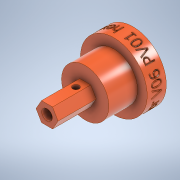
# Autodesk Inventor part: hexBushingForConnectorPiece
Saved by Autodesk Inventor 2022.2 (Build 262287000, 287)
## iProperties
Created: 2020-11-16
Part Number: hexBushingForConnectorPiece
Material: PC/ABS Plastic
Document SubType Name: Modeling
Designer: robst
Density: 0.357273 g/cm^3
Appearance: Smooth - Light Orange
Author: robst
Autodesk Inventor part; units mm, degrees
ref_plane "YZ Plane" through (0, 0, 0) normal (1, 0, 0) x (0, 1, 0)
ref_plane "XY Plane" through (0, 0, 0) normal (0, 0, 1) x (1, 0, 0)
sketch "Sketch1" plane through (0, 0, 0) normal (0, 0, 1) x (1, 0, 0)
  line L0 (7.3323, 0) -> (3.6662, -6.35)
  line L1 (3.6662, -6.35) -> (-3.6662, -6.35)
  line L2 (-3.6662, -6.35) -> (-7.3323, 0)
  line L3 (-7.3323, 0) -> (-3.6662, 6.35)
  line L4 (-3.6662, 6.35) -> (3.6662, 6.35)
  line L5 (3.6662, 6.35) -> (7.3323, 0)
  point P0 (0, 0)
  point P1 (0, 0)
  dimension "d0" = 12.7
  constraints: 12 end point, 1 coincident, 1 horizontal, 13 other
  measures "d0" distance between parallel lines of L1 L4
extrude "Extrusion1" add sketch "Sketch1" along normal mid plane 25.4
sketch "Sketch2" plane through (0, 0, -12.7) normal (0, 0, -1) x (-1, 0, 0)
  circle A0 centre (0, 0) radius 15.748
  dimension "d3" = 31.496
  constraints: 1 centre point, 1 coincident
  measures "d3" diameter of A0
extrude "Extrusion2" add sketch "Sketch2" along normal blind 19.05
sketch "Sketch3" plane through (0, 0, -31.75) normal (0, 0, -1) x (-1, 0, 0)
  circle A0 centre (0, 0) radius 22.225
  dimension "d6" = 44.45
  constraints: 1 centre point, 1 coincident
  measures "d6" diameter of A0
extrude "Extrusion3" add sketch "Sketch3" along normal blind 12.7
sketch "Sketch6" plane through (-3.6662, 6.35, 12.7) normal (0, 1, 0) x (1, 0, 0)
  line L0 (7.3323, 0) -> (0, 0) construction
  line L1 (3.6662, 0) -> (3.6662, 34.6111) construction
  line L2 (19.4142, 25.4) -> (-12.0818, 25.4) projected
  point P0 (3.6662, 12.7)
  point P1 (3.6662, 19.2024)
  dimension "d13" = 6.1976
  constraints: 2 end point, 1 midpoint, 1 point on line, 1 vertical
  measures "d13" distance from line of point (3.666, 19.202) L2
hole "Hole1" at (0, 6.35, -6.5024) direction (0, -1, 0) diameter 4.318 end through all clearance for "Hex Machine Screw" size "#6" standard "Ansi Unified Screw Threads"
sketch "Sketch7" plane through (0, 0, 12.7) normal (0, 0, 1) x (1, 0, 0)
  point P0 (0, 0)
  point P1 (0, 0)
  constraints: 1 coincident
hole "Hole2" at (0, 0, 12.7) direction (0, 0, -1) diameter 6.3246 depth 7.874 counterbore diameter 7.0891 counterbore depth 6.1239
ref_plane "Work Plane1" through (0, -22.225, -31.75) normal (0, 1, 0) x (-1, 0, 0)
sketch "Sketch8" plane through (0, -22.225, -31.75) normal (0, 1, 0) x (-1, 0, 0)
  line L0 (-22.225, -12.7) -> (22.225, -12.7) projected
  line L1 (-22.225, 0) -> (22.225, 0) projected
  line L2 (22.225, 0) -> (22.225, -12.7) construction
  line L3 (22.225, -6.35) -> (-22.225, -6.35) construction
  line L4 (-22.225, 0) -> (-22.225, -12.7) construction
  line L5 (63.482, -9.525) -> (64.2847, -9.525)
  line L6 (64.2847, -9.525) -> (64.2847, -6.808)
  spline S0 degree 2 poles (64.2847, -6.808) (64.2847, -6.4786) (64.3465, -5.9126) (64.4391, -5.7428) knots 0 0 0 1 2 2 2
  spline S1 degree 2 poles (64.4391, -5.7428) (64.5369, -5.5627) (64.8868, -5.3877) (65.1853, -5.3877) knots 0 0 0 1 2 2 2
  spline S2 degree 2 poles (65.1853, -5.3877) (65.4837, -5.3877) (66.1167, -5.7068) (66.4203, -5.9641) knots 0 0 0 1 2 2 2
  line L7 (66.4203, -5.9641) -> (66.4203, -9.525)
  line L8 (66.4203, -9.525) -> (67.223, -9.525)
  line L9 (67.223, -9.525) -> (67.223, -2.892)
  line L10 (67.223, -2.892) -> (66.4203, -2.892)
  line L11 (66.4203, -2.892) -> (66.4203, -5.29)
  spline S3 degree 2 poles (66.4203, -5.29) (66.0601, -4.9658) (65.3654, -4.6261) (64.9743, -4.6261) knots 0 0 0 1 2 2 2
  spline S4 degree 2 poles (64.9743, -4.6261) (64.2744, -4.6261) (63.482, -5.5524) (63.482, -6.4323) knots 0 0 0 1 2 2 2
  line L12 (63.482, -6.4323) -> (63.482, -9.525)
  spline S5 degree 2 poles (60.2864, -9.6331) (61.4288, -9.6331) (62.6844, -8.3517) (62.6844, -7.1682) knots 0 0 0 1 2 2 2
  spline S6 degree 2 poles (62.6844, -7.1682) (62.6844, -6.0052) (61.4648, -4.6261) (60.4819, -4.6261) knots 0 0 0 1 2 2 2
  spline S7 degree 2 poles (60.4819, -4.6261) (60.0394, -4.6261) (59.355, -4.8834) (59.1029, -5.1562) knots 0 0 0 1 2 2 2
  spline S8 degree 2 poles (59.1029, -5.1562) (58.8456, -5.4289) (58.5728, -6.2162) (58.5728, -6.7874) knots 0 0 0 1 2 2 2
  line L13 (58.5728, -6.7874) -> (58.5728, -7.2248)
  line L14 (58.5728, -7.2248) -> (61.8713, -7.2248)
  spline S9 degree 2 poles (61.8713, -7.2248) (61.8713, -8.0533) (61.0377, -8.9332) (60.2967, -8.9332) knots 0 0 0 1 2 2 2
  spline S10 degree 2 poles (60.2967, -8.9332) (60.0343, -8.9332) (59.5248, -8.8149) (59.319, -8.7222) knots 0 0 0 1 2 2 2
  spline S11 degree 2 poles (59.319, -8.7222) (59.1029, -8.6193) (58.8044, -8.4392) (58.7066, -8.3569) knots 0 0 0 1 2 2 2
  line L15 (58.7066, -8.3569) -> (58.6603, -8.3569)
  line L16 (58.6603, -8.3569) -> (58.6603, -9.2317)
  spline S12 degree 2 poles (58.6603, -9.2317) (58.7992, -9.2883) (59.2212, -9.453) (59.3859, -9.4993) knots 0 0 0 1 2 2 2
  spline S13 degree 2 poles (59.3859, -9.4993) (59.6174, -9.5662) (59.9982, -9.6331) (60.2864, -9.6331) knots 0 0 0 1 2 2 2
  spline S14 degree 2 poles (59.355, -6.6124) (59.3653, -6.2882) (59.4991, -5.8148) (59.6277, -5.6553) knots 0 0 0 1 2 2 2
  spline S15 degree 2 poles (59.6277, -5.6553) (59.7667, -5.4752) (60.2041, -5.2848) (60.5283, -5.2848) knots 0 0 0 1 2 2 2
  spline S16 degree 2 poles (60.5283, -5.2848) (60.8473, -5.2848) (61.295, -5.4752) (61.4802, -5.6605) knots 0 0 0 1 2 2 2
  spline S17 degree 2 poles (61.4802, -5.6605) (61.6603, -5.8509) (61.8456, -6.3088) (61.8713, -6.6124) knots 0 0 0 1 2 2 2
  line L17 (61.8713, -6.6124) -> (59.355, -6.6124)
  line L18 (54.0599, -9.525) -> (55.0428, -9.525)
  line L19 (55.0428, -9.525) -> (56.2006, -7.7342)
  line L20 (56.2006, -7.7342) -> (57.3893, -9.525)
  line L21 (57.3893, -9.525) -> (58.3001, -9.525)
  line L22 (58.3001, -9.525) -> (56.6483, -7.163)
  line L23 (56.6483, -7.163) -> (58.2847, -4.7599)
  line L24 (58.2847, -4.7599) -> (57.3018, -4.7599)
  line L25 (57.3018, -4.7599) -> (56.1491, -6.5353)
  line L26 (56.1491, -6.5353) -> (54.9707, -4.7599)
  line L27 (54.9707, -4.7599) -> (54.0599, -4.7599)
  line L28 (54.0599, -4.7599) -> (55.7014, -7.1116)
  line L29 (55.7014, -7.1116) -> (54.0599, -9.525)
  spline S18 degree 2 poles (49.0684, -7.5747) (49.0684, -8.0481) (49.4286, -8.7737) (49.7271, -9.0104) knots 0 0 0 1 2 2 2
  spline S19 degree 2 poles (49.7271, -9.0104) (50.0873, -9.2883) (50.9055, -9.525) (51.5539, -9.525) knots 0 0 0 1 2 2 2
  line L30 (51.5539, -9.525) -> (53.3755, -9.525)
  line L31 (53.3755, -9.525) -> (53.3755, -3.175)
  line L32 (53.3755, -3.175) -> (51.6928, -3.175)
  spline S20 degree 2 poles (51.6928, -3.175) (51.0135, -3.175) (50.3343, -3.2625) (50.0255, -3.4323) knots 0 0 0 1 2 2 2
  spline S21 degree 2 poles (50.0255, -3.4323) (49.6808, -3.6124) (49.3669, -4.2042) (49.3669, -4.6056) knots 0 0 0 1 2 2 2
  spline S22 degree 2 poles (49.3669, -4.6056) (49.3669, -5.0532) (49.8403, -5.7634) (50.2571, -5.9641) knots 0 0 0 1 2 2 2
  line L33 (50.2571, -5.9641) -> (50.2571, -5.9949)
  spline S23 degree 2 poles (50.2571, -5.9949) (49.6911, -6.1493) (49.0684, -6.9675) (49.0684, -7.5747) knots 0 0 0 1 2 2 2
  spline S24 degree 2 poles (49.9484, -7.6107) (49.9484, -7.2505) (50.1542, -6.7874) (50.4629, -6.6227) knots 0 0 0 1 2 2 2
  spline S25 degree 2 poles (50.4629, -6.6227) (50.6636, -6.5198) (51.1371, -6.4581) (51.5744, -6.4581) knots 0 0 0 1 2 2 2
  line L34 (51.5744, -6.4581) -> (52.5316, -6.4581)
  line L35 (52.5316, -6.4581) -> (52.5316, -8.8046)
  line L36 (52.5316, -8.8046) -> (51.8472, -8.8046)
  spline S26 degree 2 poles (51.8472, -8.8046) (51.2914, -8.8046) (50.6533, -8.7017) (50.4063, -8.537) knots 0 0 0 1 2 2 2
  spline S27 degree 2 poles (50.4063, -8.537) (50.1696, -8.3672) (49.9484, -7.9452) (49.9484, -7.6107) knots 0 0 0 1 2 2 2
  spline S28 degree 2 poles (50.2468, -4.7239) (50.2468, -4.4975) (50.4012, -4.1579) (50.571, -4.0601) knots 0 0 0 1 2 2 2
  spline S29 degree 2 poles (50.571, -4.0601) (50.7768, -3.9469) (51.276, -3.8954) (51.7237, -3.8954) knots 0 0 0 1 2 2 2
  line L37 (51.7237, -3.8954) -> (52.5316, -3.8954)
  line L38 (52.5316, -3.8954) -> (52.5316, -5.7531)
  line L39 (52.5316, -5.7531) -> (51.5744, -5.7531)
  spline S30 degree 2 poles (51.5744, -5.7531) (51.1782, -5.7531) (50.8026, -5.6707) (50.6019, -5.5421) knots 0 0 0 1 2 2 2
  spline S31 degree 2 poles (50.6019, -5.5421) (50.4063, -5.4186) (50.2468, -5.0224) (50.2468, -4.7239) knots 0 0 0 1 2 2 2
  line L40 (44.5864, -9.525) -> (45.3891, -9.525)
  line L41 (45.3891, -9.525) -> (45.3891, -9.0001)
  spline S32 degree 2 poles (45.3891, -9.0001) (45.7596, -9.3243) (46.4234, -9.6588) (46.8351, -9.6588) knots 0 0 0 1 2 2 2
  spline S33 degree 2 poles (46.8351, -9.6588) (47.1439, -9.6588) (47.6945, -9.453) (47.8952, -9.2317) knots 0 0 0 1 2 2 2
  spline S34 degree 2 poles (47.8952, -9.2317) (48.101, -9.0104) (48.3274, -8.3363) (48.3274, -7.8526) knots 0 0 0 1 2 2 2
  line L42 (48.3274, -7.8526) -> (48.3274, -4.7599)
  line L43 (48.3274, -4.7599) -> (47.5247, -4.7599)
  line L44 (47.5247, -4.7599) -> (47.5247, -7.4769)
  spline S35 degree 2 poles (47.5247, -7.4769) (47.5247, -7.8577) (47.468, -8.3569) (47.3703, -8.5421) knots 0 0 0 1 2 2 2
  spline S36 degree 2 poles (47.3703, -8.5421) (47.2725, -8.7274) (46.938, -8.8972) (46.6241, -8.8972) knots 0 0 0 1 2 2 2
  spline S37 degree 2 poles (46.6241, -8.8972) (46.3308, -8.8972) (45.667, -8.5627) (45.3891, -8.3209) knots 0 0 0 1 2 2 2
  line L45 (45.3891, -8.3209) -> (45.3891, -4.7599)
  line L46 (45.3891, -4.7599) -> (44.5864, -4.7599)
  line L47 (44.5864, -4.7599) -> (44.5864, -9.525)
  spline S38 degree 2 poles (42.1369, -9.6382) (42.6155, -9.6382) (43.444, -9.3809) (43.7167, -9.2368) knots 0 0 0 1 2 2 2
  line L48 (43.7167, -9.2368) -> (43.7167, -8.3363)
  line L49 (43.7167, -8.3363) -> (43.6755, -8.3363)
  spline S39 degree 2 poles (43.6755, -8.3363) (43.5726, -8.4186) (43.2947, -8.6142) (43.0632, -8.7222) knots 0 0 0 1 2 2 2
  spline S40 degree 2 poles (43.0632, -8.7222) (42.8625, -8.82) (42.3685, -8.9641) (42.1061, -8.9641) knots 0 0 0 1 2 2 2
  spline S41 degree 2 poles (42.1061, -8.9641) (41.9157, -8.9641) (41.4783, -8.8766) (41.3753, -8.8046) knots 0 0 0 1 2 2 2
  spline S42 degree 2 poles (41.3753, -8.8046) (41.2261, -8.7068) (41.0923, -8.4855) (41.0923, -8.2591) knots 0 0 0 1 2 2 2
  spline S43 degree 2 poles (41.0923, -8.2591) (41.0923, -7.9761) (41.4011, -7.6828) (41.7973, -7.585) knots 0 0 0 1 2 2 2
  spline S44 degree 2 poles (41.7973, -7.585) (41.9517, -7.549) (42.4457, -7.4461) (42.6567, -7.3895) knots 0 0 0 1 2 2 2
  spline S45 degree 2 poles (42.6567, -7.3895) (43.2021, -7.2299) (43.6961, -6.5713) (43.6961, -6.103) knots 0 0 0 1 2 2 2
  spline S46 degree 2 poles (43.6961, -6.103) (43.6961, -5.4546) (42.7236, -4.6467) (41.9208, -4.6467) knots 0 0 0 1 2 2 2
  spline S47 degree 2 poles (41.9208, -4.6467) (41.5246, -4.6467) (40.7218, -4.8423) (40.4491, -4.9915) knots 0 0 0 1 2 2 2
  line L50 (40.4491, -4.9915) -> (40.4491, -5.8509)
  line L51 (40.4491, -5.8509) -> (40.4903, -5.8509)
  spline S48 degree 2 poles (40.4903, -5.8509) (40.799, -5.6038) (41.5503, -5.3208) (41.9362, -5.3208) knots 0 0 0 1 2 2 2
  spline S49 degree 2 poles (41.9362, -5.3208) (42.3325, -5.3208) (42.8779, -5.6553) (42.8779, -5.9898) knots 0 0 0 1 2 2 2
  spline S50 degree 2 poles (42.8779, -5.9898) (42.8779, -6.2934) (42.5537, -6.5867) (42.1935, -6.6793) knots 0 0 0 1 2 2 2
  spline S51 degree 2 poles (42.1935, -6.6793) (42.0186, -6.7256) (41.576, -6.8183) (41.3342, -6.8749) knots 0 0 0 1 2 2 2
  spline S52 degree 2 poles (41.3342, -6.8749) (40.8093, -7.0087) (40.2741, -7.621) (40.2741, -8.1511) knots 0 0 0 1 2 2 2
  spline S53 degree 2 poles (40.2741, -8.1511) (40.2741, -8.4598) (40.516, -9.0053) (40.7527, -9.206) knots 0 0 0 1 2 2 2
  spline S54 degree 2 poles (40.7527, -9.206) (41.0048, -9.4169) (41.6481, -9.6382) (42.1369, -9.6382) knots 0 0 0 1 2 2 2
  line L52 (35.7869, -9.525) -> (36.5897, -9.525)
  line L53 (36.5897, -9.525) -> (36.5897, -6.808)
  spline S55 degree 2 poles (36.5897, -6.808) (36.5897, -6.4786) (36.6514, -5.9126) (36.7441, -5.7428) knots 0 0 0 1 2 2 2
  spline S56 degree 2 poles (36.7441, -5.7428) (36.8418, -5.5627) (37.1918, -5.3877) (37.4902, -5.3877) knots 0 0 0 1 2 2 2
  spline S57 degree 2 poles (37.4902, -5.3877) (37.7887, -5.3877) (38.4216, -5.7068) (38.7252, -5.9641) knots 0 0 0 1 2 2 2
  line L54 (38.7252, -5.9641) -> (38.7252, -9.525)
  line L55 (38.7252, -9.525) -> (39.528, -9.525)
  line L56 (39.528, -9.525) -> (39.528, -2.892)
  line L57 (39.528, -2.892) -> (38.7252, -2.892)
  line L58 (38.7252, -2.892) -> (38.7252, -5.29)
  spline S58 degree 2 poles (38.7252, -5.29) (38.365, -4.9658) (37.6703, -4.6261) (37.2792, -4.6261) knots 0 0 0 1 2 2 2
  spline S59 degree 2 poles (37.2792, -4.6261) (36.5794, -4.6261) (35.7869, -5.5524) (35.7869, -6.4323) knots 0 0 0 1 2 2 2
  line L59 (35.7869, -6.4323) -> (35.7869, -9.525)
  line L60 (33.8418, -9.525) -> (34.6445, -9.525)
  line L61 (34.6445, -9.525) -> (34.6445, -4.7599)
  line L62 (34.6445, -4.7599) -> (33.8418, -4.7599)
  line L63 (33.8418, -4.7599) -> (33.8418, -9.525)
  line L64 (33.7852, -3.9675) -> (34.696, -3.9675)
  line L65 (34.696, -3.9675) -> (34.696, -3.1338)
  line L66 (34.696, -3.1338) -> (33.7852, -3.1338)
  line L67 (33.7852, -3.1338) -> (33.7852, -3.9675)
  line L68 (28.9223, -9.525) -> (29.7251, -9.525)
  line L69 (29.7251, -9.525) -> (29.7251, -6.808)
  spline S60 degree 2 poles (29.7251, -6.808) (29.7251, -6.4786) (29.7868, -5.9126) (29.8795, -5.7428) knots 0 0 0 1 2 2 2
  spline S61 degree 2 poles (29.8795, -5.7428) (29.9772, -5.5627) (30.3272, -5.3877) (30.6256, -5.3877) knots 0 0 0 1 2 2 2
  spline S62 degree 2 poles (30.6256, -5.3877) (30.9241, -5.3877) (31.557, -5.7068) (31.8606, -5.9641) knots 0 0 0 1 2 2 2
  line L70 (31.8606, -5.9641) -> (31.8606, -9.525)
  line L71 (31.8606, -9.525) -> (32.6634, -9.525)
  line L72 (32.6634, -9.525) -> (32.6634, -4.7599)
  line L73 (32.6634, -4.7599) -> (31.8606, -4.7599)
  line L74 (31.8606, -4.7599) -> (31.8606, -5.29)
  spline S63 degree 2 poles (31.8606, -5.29) (31.5004, -4.9658) (30.8057, -4.6261) (30.4146, -4.6261) knots 0 0 0 1 2 2 2
  spline S64 degree 2 poles (30.4146, -4.6261) (29.7148, -4.6261) (28.9223, -5.5524) (28.9223, -6.4323) knots 0 0 0 1 2 2 2
  line L75 (28.9223, -6.4323) -> (28.9223, -9.525)
  spline S65 degree 2 poles (27.6256, -10.2866) (27.5433, -10.3226) (27.2294, -10.4358) (27.0287, -10.4821) knots 0 0 0 1 2 2 2
  spline S66 degree 2 poles (27.0287, -10.4821) (26.8074, -10.5387) (26.4317, -10.6056) (26.2105, -10.6056) knots 0 0 0 1 2 2 2
  spline S67 degree 2 poles (26.2105, -10.6056) (25.84, -10.6056) (25.3254, -10.4101) (25.1813, -10.2351) knots 0 0 0 1 2 2 2
  spline S68 degree 2 poles (25.1813, -10.2351) (25.0424, -10.0602) (24.9343, -9.6022) (24.9343, -9.3089) knots 0 0 0 1 2 2 2
  line L76 (24.9343, -9.3089) -> (24.9343, -8.8921)
  spline S69 degree 2 poles (24.9343, -8.8921) (25.2585, -9.1751) (25.8811, -9.4427) (26.3494, -9.4427) knots 0 0 0 1 2 2 2
  spline S70 degree 2 poles (26.3494, -9.4427) (27.1625, -9.4427) (28.1247, -8.2334) (28.1247, -7.0962) knots 0 0 0 1 2 2 2
  spline S71 degree 2 poles (28.1247, -7.0962) (28.1247, -6.5044) (27.7903, -5.5884) (27.5124, -5.2642) knots 0 0 0 1 2 2 2
  spline S72 degree 2 poles (27.5124, -5.2642) (27.2448, -4.9606) (26.5089, -4.6261) (26.1178, -4.6261) knots 0 0 0 1 2 2 2
  spline S73 degree 2 poles (26.1178, -4.6261) (25.7473, -4.6261) (25.207, -4.8011) (24.9343, -4.9606) knots 0 0 0 1 2 2 2
  line L77 (24.9343, -4.9606) -> (24.888, -4.7599)
  line L78 (24.888, -4.7599) -> (24.1315, -4.7599)
  line L79 (24.1315, -4.7599) -> (24.1315, -8.9795)
  spline S74 degree 2 poles (24.1315, -8.9795) (24.1315, -10.194) (25.1864, -11.3261) (26.2722, -11.3261) knots 0 0 0 1 2 2 2
  spline S75 degree 2 poles (26.2722, -11.3261) (26.6221, -11.3261) (27.3529, -11.2128) (27.6668, -11.1202) knots 0 0 0 1 2 2 2
  line L80 (27.6668, -11.1202) -> (27.6668, -10.2866)
  line L81 (27.6668, -10.2866) -> (27.6256, -10.2866)
  line L82 (24.9343, -8.2334) -> (24.9343, -5.6141)
  spline S76 degree 2 poles (24.9343, -5.6141) (25.2328, -5.4701) (25.7371, -5.3466) (25.9892, -5.3466) knots 0 0 0 1 2 2 2
  spline S77 degree 2 poles (25.9892, -5.3466) (26.5964, -5.3466) (27.2962, -6.2419) (27.2962, -7.0807) knots 0 0 0 1 2 2 2
  spline S78 degree 2 poles (27.2962, -7.0807) (27.2962, -7.8732) (26.7662, -8.7017) (26.1693, -8.7017) knots 0 0 0 1 2 2 2
  spline S79 degree 2 poles (26.1693, -8.7017) (25.8554, -8.7017) (25.1967, -8.4547) (24.9343, -8.2334) knots 0 0 0 1 2 2 2
  line L83 (19.1092, -3.9263) -> (22.0629, -3.9263)
  line L84 (22.0629, -3.9263) -> (22.0629, -5.7171)
  line L85 (22.0629, -5.7171) -> (19.2327, -5.7171)
  line L86 (19.2327, -5.7171) -> (19.2327, -6.4684)
  line L87 (19.2327, -6.4684) -> (22.0629, -6.4684)
  line L88 (22.0629, -6.4684) -> (22.0629, -9.525)
  line L89 (22.0629, -9.525) -> (22.9068, -9.525)
  line L90 (22.9068, -9.525) -> (22.9068, -3.175)
  line L91 (22.9068, -3.175) -> (19.1092, -3.175)
  line L92 (19.1092, -3.175) -> (19.1092, -3.9263)
  spline S80 degree 2 poles (14.4985, -7.1425) (14.4985, -8.3466) (15.6563, -9.6588) (16.6237, -9.6588) knots 0 0 0 1 2 2 2
  spline S81 degree 2 poles (16.6237, -9.6588) (17.6169, -9.6588) (18.7541, -8.3054) (18.7541, -7.1425) knots 0 0 0 1 2 2 2
  spline S82 degree 2 poles (18.7541, -7.1425) (18.7541, -5.9486) (17.5809, -4.6261) (16.6237, -4.6261) knots 0 0 0 1 2 2 2
  spline S83 degree 2 poles (16.6237, -4.6261) (15.6563, -4.6261) (14.4985, -5.9435) (14.4985, -7.1425) knots 0 0 0 1 2 2 2
  spline S84 degree 2 poles (15.327, -7.1425) (15.327, -6.2162) (16.0011, -5.3157) (16.6237, -5.3157) knots 0 0 0 1 2 2 2
  spline S85 degree 2 poles (16.6237, -5.3157) (17.2464, -5.3157) (17.9256, -6.2162) (17.9256, -7.1425) knots 0 0 0 1 2 2 2
  spline S86 degree 2 poles (17.9256, -7.1425) (17.9256, -8.043) (17.2464, -8.9692) (16.6237, -8.9692) knots 0 0 0 1 2 2 2
  spline S87 degree 2 poles (16.6237, -8.9692) (16.0062, -8.9692) (15.327, -8.0584) (15.327, -7.1425) knots 0 0 0 1 2 2 2
  line L93 (11.1485, -5.6193) -> (11.1897, -5.6193)
  spline S88 degree 2 poles (11.1897, -5.6193) (11.2823, -5.5936) (11.483, -5.5833) (11.6219, -5.5833) knots 0 0 0 1 2 2 2
  spline S89 degree 2 poles (11.6219, -5.5833) (11.9461, -5.5833) (12.5842, -5.8663) (12.8724, -6.1442) knots 0 0 0 1 2 2 2
  line L94 (12.8724, -6.1442) -> (12.8724, -9.525)
  line L95 (12.8724, -9.525) -> (13.6751, -9.525)
  line L96 (13.6751, -9.525) -> (13.6751, -4.7599)
  line L97 (13.6751, -4.7599) -> (12.8724, -4.7599)
  line L98 (12.8724, -4.7599) -> (12.8724, -5.4701)
  spline S90 degree 2 poles (12.8724, -5.4701) (12.435, -5.079) (11.7815, -4.7599) (11.4727, -4.7599) knots 0 0 0 1 2 2 2
  spline S91 degree 2 poles (11.4727, -4.7599) (11.3492, -4.7599) (11.2257, -4.7702) (11.1485, -4.7857) knots 0 0 0 1 2 2 2
  line L99 (11.1485, -4.7857) -> (11.1485, -5.6193)
  spline S92 degree 2 poles (7.9838, -9.6382) (8.6013, -9.6382) (9.6459, -9.2214) (10.0267, -8.8046) knots 0 0 0 1 2 2 2
  spline S93 degree 2 poles (10.0267, -8.8046) (10.4075, -8.3929) (10.8243, -7.1579) (10.8243, -6.3551) knots 0 0 0 1 2 2 2
  spline S94 degree 2 poles (10.8243, -6.3551) (10.8243, -5.5575) (10.4178, -4.374) (10.0319, -3.9366) knots 0 0 0 1 2 2 2
  spline S95 degree 2 poles (10.0319, -3.9366) (9.6511, -3.5095) (8.6116, -3.0618) (7.9684, -3.0618) knots 0 0 0 1 2 2 2
  spline S96 degree 2 poles (7.9684, -3.0618) (7.6493, -3.0618) (7.0884, -3.1544) (6.8517, -3.2265) knots 0 0 0 1 2 2 2
  spline S97 degree 2 poles (6.8517, -3.2265) (6.6459, -3.2934) (6.2188, -3.4838) (6.0078, -3.597) knots 0 0 0 1 2 2 2
  line L100 (6.0078, -3.597) -> (6.0078, -4.6158)
  line L101 (6.0078, -4.6158) -> (6.0747, -4.6158)
  spline S98 degree 2 poles (6.0747, -4.6158) (6.1879, -4.5129) (6.5378, -4.2248) (6.79, -4.0858) knots 0 0 0 1 2 2 2
  spline S99 degree 2 poles (6.79, -4.0858) (7.0318, -3.952) (7.603, -3.7822) (7.9735, -3.7822) knots 0 0 0 1 2 2 2
  spline S100 degree 2 poles (7.9735, -3.7822) (8.38, -3.7822) (9.1056, -4.1167) (9.3783, -4.4357) knots 0 0 0 1 2 2 2
  spline S101 degree 2 poles (9.3783, -4.4357) (9.6459, -4.7599) (9.9444, -5.7428) (9.9444, -6.3551) knots 0 0 0 1 2 2 2
  spline S102 degree 2 poles (9.9444, -6.3551) (9.9444, -7.0087) (9.6305, -7.9504) (9.3578, -8.2746) knots 0 0 0 1 2 2 2
  spline S103 degree 2 poles (9.3578, -8.2746) (9.0902, -8.5885) (8.3749, -8.9075) (7.9735, -8.9075) knots 0 0 0 1 2 2 2
  spline S104 degree 2 poles (7.9735, -8.9075) (7.6082, -8.9075) (6.9855, -8.7274) (6.7437, -8.5936) knots 0 0 0 1 2 2 2
  spline S105 degree 2 poles (6.7437, -8.5936) (6.5121, -8.4598) (6.1673, -8.1819) (6.0695, -8.0842) knots 0 0 0 1 2 2 2
  line L102 (6.0695, -8.0842) -> (6.0078, -8.0842)
  line L103 (6.0078, -8.0842) -> (6.0078, -9.0927)
  spline S106 degree 2 poles (6.0078, -9.0927) (6.2188, -9.1905) (6.5893, -9.3706) (6.8517, -9.453) knots 0 0 0 1 2 2 2
  spline S107 degree 2 poles (6.8517, -9.453) (7.1296, -9.5456) (7.603, -9.6382) (7.9838, -9.6382) knots 0 0 0 1 2 2 2
  spline S108 degree 2 poles (1.3662, -7.1425) (1.3662, -8.3466) (2.524, -9.6588) (3.4915, -9.6588) knots 0 0 0 1 2 2 2
  spline S109 degree 2 poles (3.4915, -9.6588) (4.4846, -9.6588) (5.6219, -8.3054) (5.6219, -7.1425) knots 0 0 0 1 2 2 2
  spline S110 degree 2 poles (5.6219, -7.1425) (5.6219, -5.9486) (4.4486, -4.6261) (3.4915, -4.6261) knots 0 0 0 1 2 2 2
  spline S111 degree 2 poles (3.4915, -4.6261) (2.524, -4.6261) (1.3662, -5.9435) (1.3662, -7.1425) knots 0 0 0 1 2 2 2
  spline S112 degree 2 poles (2.1947, -7.1425) (2.1947, -6.2162) (2.8688, -5.3157) (3.4915, -5.3157) knots 0 0 0 1 2 2 2
  spline S113 degree 2 poles (3.4915, -5.3157) (4.1141, -5.3157) (4.7934, -6.2162) (4.7934, -7.1425) knots 0 0 0 1 2 2 2
  spline S114 degree 2 poles (4.7934, -7.1425) (4.7934, -8.043) (4.1141, -8.9692) (3.4915, -8.9692) knots 0 0 0 1 2 2 2
  spline S115 degree 2 poles (3.4915, -8.9692) (2.874, -8.9692) (2.1947, -8.0584) (2.1947, -7.1425) knots 0 0 0 1 2 2 2
  line L104 (-3.1982, -9.525) -> (-2.3954, -9.525)
  line L105 (-2.3954, -9.525) -> (-2.3954, -6.808)
  spline S116 degree 2 poles (-2.3954, -6.808) (-2.3954, -6.4786) (-2.3337, -5.9126) (-2.241, -5.7428) knots 0 0 0 1 2 2 2
  spline S117 degree 2 poles (-2.241, -5.7428) (-2.1433, -5.5627) (-1.7933, -5.3877) (-1.4949, -5.3877) knots 0 0 0 1 2 2 2
  spline S118 degree 2 poles (-1.4949, -5.3877) (-1.1964, -5.3877) (-0.5635, -5.7068) (-0.2599, -5.9641) knots 0 0 0 1 2 2 2
  line L106 (-0.2599, -5.9641) -> (-0.2599, -9.525)
  line L107 (-0.2599, -9.525) -> (0.5429, -9.525)
  line L108 (0.5429, -9.525) -> (0.5429, -4.7599)
  line L109 (0.5429, -4.7599) -> (-0.2599, -4.7599)
  line L110 (-0.2599, -4.7599) -> (-0.2599, -5.29)
  spline S119 degree 2 poles (-0.2599, -5.29) (-0.6201, -4.9658) (-1.3148, -4.6261) (-1.7059, -4.6261) knots 0 0 0 1 2 2 2
  spline S120 degree 2 poles (-1.7059, -4.6261) (-2.4057, -4.6261) (-3.1982, -5.5524) (-3.1982, -6.4323) knots 0 0 0 1 2 2 2
  line L111 (-3.1982, -6.4323) -> (-3.1982, -9.525)
  line L112 (-8.0661, -9.525) -> (-7.2634, -9.525)
  line L113 (-7.2634, -9.525) -> (-7.2634, -6.808)
  spline S121 degree 2 poles (-7.2634, -6.808) (-7.2634, -6.4786) (-7.2016, -5.9126) (-7.109, -5.7428) knots 0 0 0 1 2 2 2
  spline S122 degree 2 poles (-7.109, -5.7428) (-7.0112, -5.5627) (-6.6613, -5.3877) (-6.3629, -5.3877) knots 0 0 0 1 2 2 2
  spline S123 degree 2 poles (-6.3629, -5.3877) (-6.0644, -5.3877) (-5.4315, -5.7068) (-5.1279, -5.9641) knots 0 0 0 1 2 2 2
  line L114 (-5.1279, -5.9641) -> (-5.1279, -9.525)
  line L115 (-5.1279, -9.525) -> (-4.3251, -9.525)
  line L116 (-4.3251, -9.525) -> (-4.3251, -4.7599)
  line L117 (-4.3251, -4.7599) -> (-5.1279, -4.7599)
  line L118 (-5.1279, -4.7599) -> (-5.1279, -5.29)
  spline S124 degree 2 poles (-5.1279, -5.29) (-5.4881, -4.9658) (-6.1828, -4.6261) (-6.5738, -4.6261) knots 0 0 0 1 2 2 2
  spline S125 degree 2 poles (-6.5738, -4.6261) (-7.2737, -4.6261) (-8.0661, -5.5524) (-8.0661, -6.4323) knots 0 0 0 1 2 2 2
  line L119 (-8.0661, -6.4323) -> (-8.0661, -9.525)
  spline S126 degree 2 poles (-11.2617, -9.6331) (-10.1193, -9.6331) (-8.8638, -8.3517) (-8.8638, -7.1682) knots 0 0 0 1 2 2 2
  spline S127 degree 2 poles (-8.8638, -7.1682) (-8.8638, -6.0052) (-10.0833, -4.6261) (-11.0662, -4.6261) knots 0 0 0 1 2 2 2
  spline S128 degree 2 poles (-11.0662, -4.6261) (-11.5087, -4.6261) (-12.1931, -4.8834) (-12.4453, -5.1562) knots 0 0 0 1 2 2 2
  spline S129 degree 2 poles (-12.4453, -5.1562) (-12.7026, -5.4289) (-12.9753, -6.2162) (-12.9753, -6.7874) knots 0 0 0 1 2 2 2
  line L120 (-12.9753, -6.7874) -> (-12.9753, -7.2248)
  line L121 (-12.9753, -7.2248) -> (-9.6768, -7.2248)
  spline S130 degree 2 poles (-9.6768, -7.2248) (-9.6768, -8.0533) (-10.5104, -8.9332) (-11.2514, -8.9332) knots 0 0 0 1 2 2 2
  spline S131 degree 2 poles (-11.2514, -8.9332) (-11.5139, -8.9332) (-12.0233, -8.8149) (-12.2292, -8.7222) knots 0 0 0 1 2 2 2
  spline S132 degree 2 poles (-12.2292, -8.7222) (-12.4453, -8.6193) (-12.7437, -8.4392) (-12.8415, -8.3569) knots 0 0 0 1 2 2 2
  line L122 (-12.8415, -8.3569) -> (-12.8878, -8.3569)
  line L123 (-12.8878, -8.3569) -> (-12.8878, -9.2317)
  spline S133 degree 2 poles (-12.8878, -9.2317) (-12.7489, -9.2883) (-12.3269, -9.453) (-12.1623, -9.4993) knots 0 0 0 1 2 2 2
  spline S134 degree 2 poles (-12.1623, -9.4993) (-11.9307, -9.5662) (-11.5499, -9.6331) (-11.2617, -9.6331) knots 0 0 0 1 2 2 2
  spline S135 degree 2 poles (-12.1931, -6.6124) (-12.1828, -6.2882) (-12.049, -5.8148) (-11.9204, -5.6553) knots 0 0 0 1 2 2 2
  spline S136 degree 2 poles (-11.9204, -5.6553) (-11.7815, -5.4752) (-11.3441, -5.2848) (-11.0199, -5.2848) knots 0 0 0 1 2 2 2
  spline S137 degree 2 poles (-11.0199, -5.2848) (-10.7008, -5.2848) (-10.2531, -5.4752) (-10.0679, -5.6605) knots 0 0 0 1 2 2 2
  spline S138 degree 2 poles (-10.0679, -5.6605) (-9.8878, -5.8509) (-9.7025, -6.3088) (-9.6768, -6.6124) knots 0 0 0 1 2 2 2
  line L124 (-9.6768, -6.6124) -> (-12.1931, -6.6124)
  spline S139 degree 2 poles (-15.682, -9.6331) (-15.188, -9.6331) (-14.3698, -9.3295) (-14.0765, -9.0207) knots 0 0 0 1 2 2 2
  spline S140 degree 2 poles (-14.0765, -9.0207) (-13.7832, -8.7171) (-13.459, -7.7806) (-13.459, -7.1528) knots 0 0 0 1 2 2 2
  spline S141 degree 2 poles (-13.459, -7.1528) (-13.459, -6.525) (-13.7935, -5.609) (-14.0765, -5.3002) knots 0 0 0 1 2 2 2
  spline S142 degree 2 poles (-14.0765, -5.3002) (-14.3595, -4.9863) (-15.1983, -4.6519) (-15.682, -4.6519) knots 0 0 0 1 2 2 2
  spline S143 degree 2 poles (-15.682, -4.6519) (-16.0731, -4.6519) (-16.8038, -4.8731) (-17.0869, -5.0172) knots 0 0 0 1 2 2 2
  line L125 (-17.0869, -5.0172) -> (-17.0869, -5.9177)
  line L126 (-17.0869, -5.9177) -> (-17.0405, -5.9177)
  spline S144 degree 2 poles (-17.0405, -5.9177) (-16.9531, -5.8457) (-16.6855, -5.6605) (-16.4951, -5.5627) knots 0 0 0 1 2 2 2
  spline S145 degree 2 poles (-16.4951, -5.5627) (-16.3253, -5.4803) (-15.8724, -5.3517) (-15.6666, -5.3517) knots 0 0 0 1 2 2 2
  spline S146 degree 2 poles (-15.6666, -5.3517) (-15.0439, -5.3517) (-14.2875, -6.2934) (-14.2875, -7.1528) knots 0 0 0 1 2 2 2
  spline S147 degree 2 poles (-14.2875, -7.1528) (-14.2875, -7.9915) (-15.0182, -8.9332) (-15.6666, -8.9332) knots 0 0 0 1 2 2 2
  spline S148 degree 2 poles (-15.6666, -8.9332) (-16.0577, -8.9332) (-16.7678, -8.609) (-17.0405, -8.3569) knots 0 0 0 1 2 2 2
  line L127 (-17.0405, -8.3569) -> (-17.0869, -8.3569)
  line L128 (-17.0869, -8.3569) -> (-17.0869, -9.2574)
  spline S149 degree 2 poles (-17.0869, -9.2574) (-16.9685, -9.314) (-16.6083, -9.4735) (-16.4642, -9.5096) knots 0 0 0 1 2 2 2
  spline S150 degree 2 poles (-16.4642, -9.5096) (-16.2584, -9.5713) (-15.9342, -9.6331) (-15.682, -9.6331) knots 0 0 0 1 2 2 2
  spline S151 degree 2 poles (-19.2584, -9.6176) (-18.6049, -9.6176) (-17.869, -8.8715) (-17.869, -8.0636) knots 0 0 0 1 2 2 2
  line L129 (-17.869, -8.0636) -> (-17.869, -5.4237)
  line L130 (-17.869, -5.4237) -> (-17.3287, -5.4237)
  line L131 (-17.3287, -5.4237) -> (-17.3287, -4.7599)
  line L132 (-17.3287, -4.7599) -> (-17.869, -4.7599)
  line L133 (-17.869, -4.7599) -> (-17.869, -3.3911)
  line L134 (-17.869, -3.3911) -> (-18.6718, -3.3911)
  line L135 (-18.6718, -3.3911) -> (-18.6718, -4.7599)
  line L136 (-18.6718, -4.7599) -> (-20.1486, -4.7599)
  line L137 (-20.1486, -4.7599) -> (-20.1486, -5.4237)
  line L138 (-20.1486, -5.4237) -> (-18.6718, -5.4237)
  line L139 (-18.6718, -5.4237) -> (-18.6718, -7.6931)
  spline S152 degree 2 poles (-18.6718, -7.6931) (-18.6718, -8.0533) (-18.6975, -8.4495) (-18.785, -8.6193) knots 0 0 0 1 2 2 2
  spline S153 degree 2 poles (-18.785, -8.6193) (-18.857, -8.7686) (-19.1812, -8.9178) (-19.4591, -8.9178) knots 0 0 0 1 2 2 2
  spline S154 degree 2 poles (-19.4591, -8.9178) (-19.6546, -8.9178) (-20.02, -8.7994) (-20.1023, -8.7634) knots 0 0 0 1 2 2 2
  line L140 (-20.1023, -8.7634) -> (-20.1486, -8.7634)
  line L141 (-20.1486, -8.7634) -> (-20.1486, -9.4838)
  spline S155 degree 2 poles (-20.1486, -9.4838) (-19.9222, -9.5456) (-19.4591, -9.6176) (-19.2584, -9.6176) knots 0 0 0 1 2 2 2
  spline S156 degree 2 poles (-24.6564, -7.1425) (-24.6564, -8.3466) (-23.4986, -9.6588) (-22.5312, -9.6588) knots 0 0 0 1 2 2 2
  spline S157 degree 2 poles (-22.5312, -9.6588) (-21.538, -9.6588) (-20.4008, -8.3054) (-20.4008, -7.1425) knots 0 0 0 1 2 2 2
  spline S158 degree 2 poles (-20.4008, -7.1425) (-20.4008, -5.9486) (-21.574, -4.6261) (-22.5312, -4.6261) knots 0 0 0 1 2 2 2
  spline S159 degree 2 poles (-22.5312, -4.6261) (-23.4986, -4.6261) (-24.6564, -5.9435) (-24.6564, -7.1425) knots 0 0 0 1 2 2 2
  spline S160 degree 2 poles (-23.8279, -7.1425) (-23.8279, -6.2162) (-23.1538, -5.3157) (-22.5312, -5.3157) knots 0 0 0 1 2 2 2
  spline S161 degree 2 poles (-22.5312, -5.3157) (-21.9085, -5.3157) (-21.2293, -6.2162) (-21.2293, -7.1425) knots 0 0 0 1 2 2 2
  spline S162 degree 2 poles (-21.2293, -7.1425) (-21.2293, -8.043) (-21.9085, -8.9692) (-22.5312, -8.9692) knots 0 0 0 1 2 2 2
  spline S163 degree 2 poles (-22.5312, -8.9692) (-23.1487, -8.9692) (-23.8279, -8.0584) (-23.8279, -7.1425) knots 0 0 0 1 2 2 2
  line L142 (-28.0064, -5.6193) -> (-27.9652, -5.6193)
  spline S164 degree 2 poles (-27.9652, -5.6193) (-27.8726, -5.5936) (-27.6719, -5.5833) (-27.533, -5.5833) knots 0 0 0 1 2 2 2
  spline S165 degree 2 poles (-27.533, -5.5833) (-27.2088, -5.5833) (-26.5707, -5.8663) (-26.2825, -6.1442) knots 0 0 0 1 2 2 2
  line L143 (-26.2825, -6.1442) -> (-26.2825, -9.525)
  line L144 (-26.2825, -9.525) -> (-25.4798, -9.525)
  line L145 (-25.4798, -9.525) -> (-25.4798, -4.7599)
  line L146 (-25.4798, -4.7599) -> (-26.2825, -4.7599)
  line L147 (-26.2825, -4.7599) -> (-26.2825, -5.4701)
  spline S166 degree 2 poles (-26.2825, -5.4701) (-26.7199, -5.079) (-27.3734, -4.7599) (-27.6822, -4.7599) knots 0 0 0 1 2 2 2
  spline S167 degree 2 poles (-27.6822, -4.7599) (-27.8057, -4.7599) (-27.9292, -4.7702) (-28.0064, -4.7857) knots 0 0 0 1 2 2 2
  line L148 (-28.0064, -4.7857) -> (-28.0064, -5.6193)
  line L149 (-36.0236, -3.175) -> (-33.8366, -9.525)
  line L150 (-33.8366, -9.525) -> (-32.9258, -9.525)
  line L151 (-32.9258, -9.525) -> (-30.7388, -3.175)
  line L152 (-30.7388, -3.175) -> (-31.6445, -3.175)
  line L153 (-31.6445, -3.175) -> (-33.4044, -8.4495)
  line L154 (-33.4044, -8.4495) -> (-35.1643, -3.175)
  line L155 (-35.1643, -3.175) -> (-36.0236, -3.175)
  spline S168 degree 2 poles (-40.4748, -6.35) (-40.4748, -8.0584) (-39.4817, -9.6588) (-38.4473, -9.6588) knots 0 0 0 1 2 2 2
  spline S169 degree 2 poles (-38.4473, -9.6588) (-37.3976, -9.6588) (-36.4147, -8.0276) (-36.4147, -6.3551) knots 0 0 0 1 2 2 2
  spline S170 degree 2 poles (-36.4147, -6.3551) (-36.4147, -4.6364) (-37.4079, -3.0464) (-38.4473, -3.0464) knots 0 0 0 1 2 2 2
  spline S171 degree 2 poles (-38.4473, -3.0464) (-39.492, -3.0464) (-40.4748, -4.693) (-40.4748, -6.35) knots 0 0 0 1 2 2 2
  spline S172 degree 2 poles (-39.3839, -8.2848) (-39.5074, -7.9709) (-39.6103, -7.0035) (-39.6103, -6.35) knots 0 0 0 1 2 2 2
  spline S173 degree 2 poles (-39.6103, -6.35) (-39.6103, -5.6965) (-39.5074, -4.7342) (-39.3787, -4.41) knots 0 0 0 1 2 2 2
  spline S174 degree 2 poles (-39.3787, -4.41) (-39.2501, -4.0858) (-38.8024, -3.7513) (-38.4473, -3.7513) knots 0 0 0 1 2 2 2
  spline S175 degree 2 poles (-38.4473, -3.7513) (-38.0923, -3.7513) (-37.6343, -4.0858) (-37.5005, -4.4203) knots 0 0 0 1 2 2 2
  spline S176 degree 2 poles (-37.5005, -4.4203) (-37.3719, -4.7445) (-37.2792, -5.7325) (-37.2792, -6.3551) knots 0 0 0 1 2 2 2
  spline S177 degree 2 poles (-37.2792, -6.3551) (-37.2792, -7.0241) (-37.3616, -7.9195) (-37.4954, -8.2694) knots 0 0 0 1 2 2 2
  spline S178 degree 2 poles (-37.4954, -8.2694) (-37.6189, -8.5987) (-38.0768, -8.9538) (-38.4473, -8.9538) knots 0 0 0 1 2 2 2
  spline S179 degree 2 poles (-38.4473, -8.9538) (-38.7973, -8.9538) (-39.2552, -8.6193) (-39.3839, -8.2848) knots 0 0 0 1 2 2 2
  spline S180 degree 2 poles (-45.3016, -7.4667) (-45.3016, -7.9555) (-44.9775, -8.784) (-44.7047, -9.0619) knots 0 0 0 1 2 2 2
  spline S181 degree 2 poles (-44.7047, -9.0619) (-44.4217, -9.3552) (-43.7116, -9.6588) (-43.2845, -9.6588) knots 0 0 0 1 2 2 2
  spline S182 degree 2 poles (-43.2845, -9.6588) (-42.8574, -9.6588) (-42.1524, -9.3706) (-41.8848, -9.0825) knots 0 0 0 1 2 2 2
  spline S183 degree 2 poles (-41.8848, -9.0825) (-41.5554, -8.7377) (-41.1849, -7.5799) (-41.1849, -6.7359) knots 0 0 0 1 2 2 2
  spline S184 degree 2 poles (-41.1849, -6.7359) (-41.1849, -5.9075) (-41.5246, -4.5747) (-41.8796, -4.0807) knots 0 0 0 1 2 2 2
  spline S185 degree 2 poles (-41.8796, -4.0807) (-42.2244, -3.597) (-43.3153, -3.0566) (-44.0306, -3.0566) knots 0 0 0 1 2 2 2
  spline S186 degree 2 poles (-44.0306, -3.0566) (-44.2416, -3.0566) (-44.6121, -3.0978) (-44.751, -3.1441) knots 0 0 0 1 2 2 2
  line L156 (-44.751, -3.1441) -> (-44.751, -3.9623)
  line L157 (-44.751, -3.9623) -> (-44.715, -3.9623)
  spline S187 degree 2 poles (-44.715, -3.9623) (-44.5967, -3.9006) (-44.1644, -3.7925) (-43.9174, -3.7925) knots 0 0 0 1 2 2 2
  spline S188 degree 2 poles (-43.9174, -3.7925) (-43.1249, -3.7925) (-42.1524, -4.8628) (-42.0597, -5.9126) knots 0 0 0 1 2 2 2
  spline S189 degree 2 poles (-42.0597, -5.9126) (-42.3634, -5.7016) (-43.0014, -5.4701) (-43.3822, -5.4701) knots 0 0 0 1 2 2 2
  spline S190 degree 2 poles (-43.3822, -5.4701) (-43.7527, -5.4701) (-44.3085, -5.6193) (-44.6121, -5.8457) knots 0 0 0 1 2 2 2
  spline S191 degree 2 poles (-44.6121, -5.8457) (-44.962, -6.1081) (-45.3016, -6.9212) (-45.3016, -7.4667) knots 0 0 0 1 2 2 2
  spline S192 degree 2 poles (-44.4371, -7.5027) (-44.4371, -7.1116) (-44.2313, -6.5816) (-44.0049, -6.3963) knots 0 0 0 1 2 2 2
  spline S193 degree 2 poles (-44.0049, -6.3963) (-43.8351, -6.2625) (-43.4131, -6.175) (-43.1918, -6.175) knots 0 0 0 1 2 2 2
  spline S194 degree 2 poles (-43.1918, -6.175) (-42.8934, -6.175) (-42.3325, -6.3551) (-42.0597, -6.525) knots 0 0 0 1 2 2 2
  spline S195 degree 2 poles (-42.0597, -6.525) (-42.0546, -6.6176) (-42.0443, -6.7925) (-42.0443, -6.9263) knots 0 0 0 1 2 2 2
  spline S196 degree 2 poles (-42.0443, -6.9263) (-42.0443, -7.585) (-42.3016, -8.3929) (-42.4971, -8.6039) knots 0 0 0 1 2 2 2
  spline S197 degree 2 poles (-42.4971, -8.6039) (-42.6772, -8.8046) (-43.0683, -8.9641) (-43.2896, -8.9641) knots 0 0 0 1 2 2 2
  spline S198 degree 2 poles (-43.2896, -8.9641) (-43.8042, -8.9641) (-44.4371, -8.2334) (-44.4371, -7.5027) knots 0 0 0 1 2 2 2
  spline S199 degree 2 poles (-52.9741, -5.0893) (-52.9741, -5.5009) (-52.6808, -6.2419) (-52.4184, -6.4992) knots 0 0 0 1 2 2 2
  spline S200 degree 2 poles (-52.4184, -6.4992) (-52.089, -6.8234) (-51.1988, -7.1579) (-50.5196, -7.1579) knots 0 0 0 1 2 2 2
  line L158 (-50.5196, -7.1579) -> (-49.8043, -7.1579)
  line L159 (-49.8043, -7.1579) -> (-49.8043, -9.525)
  line L160 (-49.8043, -9.525) -> (-48.9604, -9.525)
  line L161 (-48.9604, -9.525) -> (-48.9604, -3.175)
  line L162 (-48.9604, -3.175) -> (-50.5556, -3.175)
  spline S201 degree 2 poles (-50.5556, -3.175) (-51.1216, -3.175) (-51.9141, -3.3603) (-52.2177, -3.5712) knots 0 0 0 1 2 2 2
  spline S202 degree 2 poles (-52.2177, -3.5712) (-52.5728, -3.8131) (-52.9741, -4.5592) (-52.9741, -5.0893) knots 0 0 0 1 2 2 2
  spline S203 degree 2 poles (-52.0942, -5.115) (-52.0942, -4.7857) (-51.8678, -4.3019) (-51.6362, -4.1476) knots 0 0 0 1 2 2 2
  spline S204 degree 2 poles (-51.6362, -4.1476) (-51.4355, -4.0138) (-50.9003, -3.9057) (-50.5041, -3.9057) knots 0 0 0 1 2 2 2
  line L163 (-50.5041, -3.9057) -> (-49.8043, -3.9057)
  line L164 (-49.8043, -3.9057) -> (-49.8043, -6.4375)
  line L165 (-49.8043, -6.4375) -> (-50.3806, -6.4375)
  spline S205 degree 2 poles (-50.3806, -6.4375) (-50.8952, -6.4375) (-51.5281, -6.2728) (-51.734, -6.0567) knots 0 0 0 1 2 2 2
  spline S206 degree 2 poles (-51.734, -6.0567) (-51.9244, -5.8663) (-52.0942, -5.4186) (-52.0942, -5.115) knots 0 0 0 1 2 2 2
  line L166 (-58.3824, -3.175) -> (-56.1954, -9.525)
  line L167 (-56.1954, -9.525) -> (-55.2846, -9.525)
  line L168 (-55.2846, -9.525) -> (-53.0976, -3.175)
  line L169 (-53.0976, -3.175) -> (-54.0033, -3.175)
  line L170 (-54.0033, -3.175) -> (-55.7632, -8.4495)
  line L171 (-55.7632, -8.4495) -> (-57.5231, -3.175)
  line L172 (-57.5231, -3.175) -> (-58.3824, -3.175)
  spline S207 degree 2 poles (-62.8336, -6.35) (-62.8336, -8.0584) (-61.8405, -9.6588) (-60.8061, -9.6588) knots 0 0 0 1 2 2 2
  spline S208 degree 2 poles (-60.8061, -9.6588) (-59.7564, -9.6588) (-58.7735, -8.0276) (-58.7735, -6.3551) knots 0 0 0 1 2 2 2
  spline S209 degree 2 poles (-58.7735, -6.3551) (-58.7735, -4.6364) (-59.7667, -3.0464) (-60.8061, -3.0464) knots 0 0 0 1 2 2 2
  spline S210 degree 2 poles (-60.8061, -3.0464) (-61.8507, -3.0464) (-62.8336, -4.693) (-62.8336, -6.35) knots 0 0 0 1 2 2 2
  spline S211 degree 2 poles (-61.7427, -8.2848) (-61.8662, -7.9709) (-61.9691, -7.0035) (-61.9691, -6.35) knots 0 0 0 1 2 2 2
  spline S212 degree 2 poles (-61.9691, -6.35) (-61.9691, -5.6965) (-61.8662, -4.7342) (-61.7375, -4.41) knots 0 0 0 1 2 2 2
  spline S213 degree 2 poles (-61.7375, -4.41) (-61.6089, -4.0858) (-61.1612, -3.7513) (-60.8061, -3.7513) knots 0 0 0 1 2 2 2
  spline S214 degree 2 poles (-60.8061, -3.7513) (-60.4511, -3.7513) (-59.9931, -4.0858) (-59.8593, -4.4203) knots 0 0 0 1 2 2 2
  spline S215 degree 2 poles (-59.8593, -4.4203) (-59.7307, -4.7445) (-59.638, -5.7325) (-59.638, -6.3551) knots 0 0 0 1 2 2 2
  spline S216 degree 2 poles (-59.638, -6.3551) (-59.638, -7.0241) (-59.7204, -7.9195) (-59.8542, -8.2694) knots 0 0 0 1 2 2 2
  spline S217 degree 2 poles (-59.8542, -8.2694) (-59.9777, -8.5987) (-60.4356, -8.9538) (-60.8061, -8.9538) knots 0 0 0 1 2 2 2
  spline S218 degree 2 poles (-60.8061, -8.9538) (-61.1561, -8.9538) (-61.614, -8.6193) (-61.7427, -8.2848) knots 0 0 0 1 2 2 2
  line L173 (-67.2436, -9.525) -> (-64.1458, -9.525)
  line L174 (-64.1458, -9.525) -> (-64.1458, -8.8766)
  line L175 (-64.1458, -8.8766) -> (-65.2985, -8.8766)
  line L176 (-65.2985, -8.8766) -> (-65.2985, -4.621)
  line L177 (-65.2985, -4.621) -> (-64.1458, -4.621)
  line L178 (-64.1458, -4.621) -> (-64.1458, -4.0395)
  spline S219 degree 2 poles (-64.1458, -4.0395) (-64.7993, -4.0395) (-65.4168, -3.669) (-65.458, -3.1544) knots 0 0 0 1 2 2 2
  line L179 (-65.458, -3.1544) -> (-66.1167, -3.1544)
  line L180 (-66.1167, -3.1544) -> (-66.1167, -8.8766)
  line L181 (-66.1167, -8.8766) -> (-67.2436, -8.8766)
  line L182 (-67.2436, -8.8766) -> (-67.2436, -9.525)
  point P0 (0, 31.75)
  constraints: 2 end point, 2 midpoint, 1 horizontal
emboss "Emboss2" sketch "Sketch8" operation cut depth 2.54 direction (0, -1, 0) wrap yes faces at (-22.1529, -1.7884, -40.2167)
equation "\"d0\" = printedHexSize"
equation "\"d1\" = lengthOfHexExtrusion"
equation "\"hexSize\" = 12.7"
equation "\"slipFitOffset\" = 0"
equation "\"printedHexSize\" = hexSize - slipFitOffset"
equation "\"lengthOfHexExtrusion\" = 25.4"
equation "\"bushingSlipOffset\" = 0.381"
body "Solid1"
